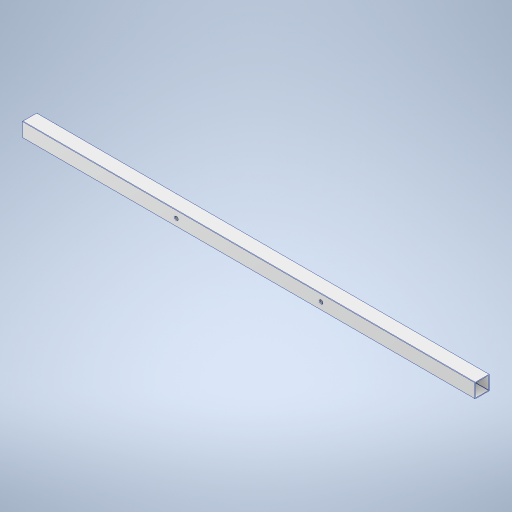
# Autodesk Inventor part: Quer_Traverse_Sitz
Saved by Autodesk Inventor 2024.4 (Build 284460000, 460)
## iProperties
Created: 2026-01-10
Part Number: Quer_Traverse_Sitz
Material: Aluminium 6061
Description: Quer_Traverse_Sitz
Document SubType Name: Modeling
Designer: julia
Mass: 1021.96 g
Surface Area: 3769.59 cm^2
Volume: 378.503 cm^3
Density: 2.7 g/cm^3
Appearance: Aluminium - flach
DocNumber: Quer_Traverse_Sitz.ipt
Folder: I60-Konstruktion\I60-Gruppe-7\Gestell\
VDS_Category: Konstruktion
Masse[kg]: 0,379 kg
Autodesk Inventor part; units mm, degrees
ref_plane "YZ Plane" through (0, 0, 0) normal (1, 0, 0) x (0, 1, 0)
ref_plane "XZ Plane" through (0, 0, 0) normal (0, 1, 0) x (-1, 0, 0)
ref_plane "XY Plane" through (0, 0, 0) normal (0, 0, 1) x (1, 0, 0)
sketch "Skizze1" plane through (0, 0, 0) normal (1, 0, 0) x (0, 1, 0)
  line L0 (-19, 20) -> (19, 20)
  line L1 (20, 19) -> (20, -19)
  line L2 (19, -20) -> (-19, -20)
  line L3 (-20, -19) -> (-20, 19)
  line L4 (-20, 20) -> (20, -20) construction
  line L5 (20, 20) -> (-20, -20) construction
  line L6 (-17.5, 18) -> (17.5, 18)
  line L7 (18, 17.5) -> (18, -17.5)
  line L8 (17.5, -18) -> (-17.5, -18)
  line L9 (-18, -17.5) -> (-18, 17.5)
  line L10 (-18, 18) -> (18, -18) construction
  line L11 (18, 18) -> (-18, -18) construction
  arc A0 (20, 19) -> (19, 20) centre (19, 19) ccw
  arc A1 (-19, 20) -> (-20, 19) centre (-19, 19) ccw
  arc A2 (-20, -19) -> (-19, -20) centre (-19, -19) ccw
  arc A3 (19, -20) -> (20, -19) centre (19, -19) ccw
  arc A4 (18, 17.5) -> (17.5, 18) centre (17.5, 17.5) ccw
  arc A5 (-17.5, 18) -> (-18, 17.5) centre (-17.5, 17.5) ccw
  arc A6 (-18, -17.5) -> (-17.5, -18) centre (-17.5, -17.5) ccw
  arc A7 (17.5, -18) -> (18, -17.5) centre (17.5, -17.5) ccw
  point P0 (0, 0)
  dimension "d0" = 40
  dimension "d1" = 40
  dimension "d2" = 36
  dimension "d3" = 36
  dimension "d4" = 1
  dimension "d5" = 0.5
  constraints: 24 end point, 16 point on circle, 16 point on line, 16 tangent, 8 centre point, 6 equal radius, 4 midpoint, 4 parallel, 2 horizontal, 2 perpendicular
  measures "d0" distance of L4.end L5.end
  measures "d1" distance of L5.start L4.end
  measures "d2" distance of L10.end L11.end
  measures "d3" distance of L11.start L10.end
  measures "d4" radius of A0
  measures "d5" radius of A4
extrude "Extrusion1" add sketch "Skizze1" along normal blind 1250
sketch "Skizze2" plane through (0, 20, 19) normal (0, 1, 0) x (1, 0, 0)
  line L0 (0, 19) -> (425, 19)
  circle A0 centre (425, 19) radius 5.25
  line L1 (425, 19) -> (825, 19)
  circle A1 centre (825, 19) radius 5.25
  dimension "d8" = 425
  dimension "d9" = 10.5
  dimension "d10" = 400
  dimension "d11" = 10.5
  constraints: 4 end point, 2 centre point, 2 coincident, 2 horizontal
  measures "d8" distance of L0.start L0.end
  measures "d9" diameter of A0
  measures "d10" distance of L1.start L1.end
  measures "d11" diameter of A1
extrude "Extrusion2" cut sketch "Skizze2" against normal blind 1250
